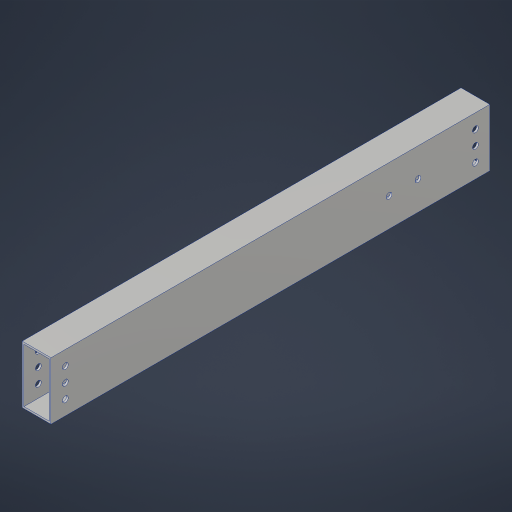
# Autodesk Inventor part: CL7-001
Saved by Autodesk Inventor 2023.4 (Build 274418000, 418)
## iProperties
RuleStatus: InUse
Created: 2025-03-17
Part Number: CL7-001
Material: Aluminum 6061
Document SubType Name: Modeling
Designer: dlangdon
Mass: 240.722 g
Surface Area: 1131.82 cm^2
Volume: 89.1563 cm^3
Density: 2.7 g/cm^3
Appearance: Aluminum - Flat
AfterDocNew0: SHOW
AfterDocOpen0: SHOW
Author: dlangdon
Autodesk Inventor part; units mm, degrees
ref_plane "YZ Plane" through (0, 0, 0) normal (1, 0, 0) x (0, 1, 0)
ref_plane "XZ Plane" through (0, 0, 0) normal (0, 1, 0) x (-1, 0, 0)
ref_plane "XY Plane" through (0, 0, 0) normal (0, 0, 1) x (1, 0, 0)
sketch "Sketch1" plane through (0, 0, 0) normal (0, 0, 1) x (1, 0, 0)
  line L0 (-12.7, -25.4) -> (12.7, -25.4)
  line L1 (12.7, -25.4) -> (12.7, 25.4)
  line L2 (12.7, 25.4) -> (-12.7, 25.4)
  line L3 (-12.7, 25.4) -> (-12.7, -25.4)
  line L4 (-12.7, -25.4) -> (12.7, 25.4) construction
  line L5 (12.7, -25.4) -> (-12.7, 25.4) construction
  line L6 (-11.1125, 23.8125) -> (11.1125, 23.8125)
  line L7 (11.1125, 23.8125) -> (11.1125, -23.8125)
  line L8 (11.1125, -23.8125) -> (-11.1125, -23.8125)
  line L9 (-11.1125, -23.8125) -> (-11.1125, 23.8125)
  point P0 (0, 0)
  dimension "width" = 25.4
  dimension "height" = 50.8
  dimension "thickness" = 1.5875
  constraints: 20 end point, 4 parallel, 2 midpoint, 2 perpendicular, 1 horizontal, 3 other
  measures "width" distance of L2.end L1.end
  measures "height" distance of L1.end L0.end
  measures "thickness" distance between parallel lines of L2 L6
extrude "Extrusion1" add sketch "Sketch1" along normal mid plane 387.35
sketch "Sketch2" plane through (12.7, -25.4, 193.675) normal (1, 0, 0) x (0, 0, -1)
  line L0 (387.35, 50.8) -> (387.35, 0) construction
  line L1 (387.35, 0) -> (0, 0) construction
  line L2 (0, 0) -> (0, 50.8) construction
  line L3 (0, 50.8) -> (387.35, 50.8) construction
  line L4 (387.35, 0) -> (0, 0) construction
  line L5 (0, 0) -> (0, 50.8) construction
  line L6 (0, 50.8) -> (387.35, 50.8) construction
  line L7 (387.35, 50.8) -> (387.35, 0) projected
  point P0 (193.675, 25.4)
  point P1 (12.7, 38.1)
  point P2 (12.7, 25.4)
  point P3 (0, 25.4)
  point P4 (12.7, 12.7)
  dimension "d5" = 12.7
  dimension "d6" = 12.7
  dimension "d7" = 12.7
  constraints: 2 vertical alignment, 1 horizontal alignment, 1 midpoint
  measures "d5" distance from line of L2 point (12.7, 25.4)
  measures "d6" distance of point (12.7, 25.4) point (12.7, 38.1)
  measures "d7" distance of point (12.7, 12.7) point (12.7, 25.4)
hole "Hole1" at (12.7, 12.7, 180.975) at (12.7, 0, 180.975) at (12.7, -12.7, 180.975) direction (-1, 0, 0) diameter 5.1054 end through all clearance for "Flat Head Machine Screw (82)" size "#10" standard "Ansi Unified Screw Threads"
mirror "Mirror1" about plane through (0, 0, 0) normal (0, 0, 1) of "Hole1"
sketch "Sketch3" plane through (12.7, -25.4, 193.675) normal (1, 0, 0) x (0, 0, -1)
  circle A0 centre (374.65, 12.7) radius 2.5527 construction
  circle A1 centre (374.65, 38.1) radius 2.5527 construction
  circle A2 centre (374.65, 25.4) radius 2.5527 construction
  circle A3 centre (12.7, 25.4) radius 2.5527 construction
  circle A4 centre (12.7, 38.1) radius 2.5527 construction
  circle A5 centre (12.7, 12.7) radius 2.5527 construction
  line L0 (387.35, 50.8) -> (387.35, 0) construction
  line L1 (387.35, 0) -> (0, 0) construction
  line L2 (0, 0) -> (0, 50.8) construction
  line L3 (0, 50.8) -> (387.35, 50.8) construction
  point P0 (193.675, 25.4)
  point P1 (323.85, 25.4)
  point P2 (298.45, 25.4)
  dimension "d15" = 50.8
  dimension "d16" = 25.4
  constraints: 2 horizontal alignment
  measures "d15" distance of point (323.85, 25.4) A2.centre
  measures "d16" distance of point (298.45, 25.4) point (323.85, 25.4)
hole "Hole2" at (12.7, 0, -130.175) at (12.7, 0, -104.775) direction (-1, 0, 0) diameter 5.1054 end through all clearance for "Flat Head Machine Screw (82)" size "#10" standard "Ansi Unified Screw Threads"
equation "\"d7\" = d6"
body "Solid1"
